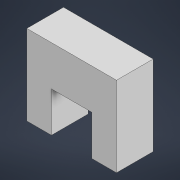
# Autodesk Inventor part: Spacer
Saved by Autodesk Inventor 2022 (Build 260153000, 153)
## iProperties
Created: 2023-04-14
Part Number: Spacer
Material: Všeobecné
Document SubType Name: Modeling
Designer: tada
Density: 1 g/cm^3
Appearance: Výchozí
Author: tada
Autodesk Inventor part; units mm, degrees
ref_plane "YZ Plane" through (0, 0, 0) normal (1, 0, 0) x (0, 1, 0)
ref_plane "XZ Plane" through (0, 0, 0) normal (0, 1, 0) x (-1, 0, 0)
ref_plane "XY Plane" through (0, 0, 0) normal (0, 0, 1) x (1, 0, 0)
sketch "Náčrt1" plane through (0, 0, 0) normal (0, 0, 1) x (1, 0, 0)
  line L0 (7.0986, 0.1592) -> (11.0986, 0.1592)
  line L1 (11.0986, 0.1592) -> (11.0986, 6.6592)
  line L2 (11.0986, 6.6592) -> (17.6486, 6.6592)
  line L3 (17.6486, 6.6592) -> (17.6486, 0.1592)
  line L4 (17.6486, 0.1592) -> (21.6486, 0.1592)
  line L5 (21.6486, 0.1592) -> (21.6486, 13.1592)
  line L6 (21.6486, 13.1592) -> (7.0986, 13.1592)
  line L7 (7.0986, 13.1592) -> (7.0986, 0.1592)
  point P0 (0, 0)
  dimension "d0" = 6.55
  dimension "d1" = 4
  dimension "d2" = 4
  dimension "d3" = 6.5
  dimension "d4" = 13
  constraints: 16 end point, 6 perpendicular, 2 point on line, 1 horizontal
  measures "d0" distance between parallel lines of L1 L3
  measures "d1" distance of L0.start L0.end
  measures "d2" distance of L3.end L4.end
  measures "d3" distance between parallel lines of L2 L0
  measures "d4" distance of L6.end L0.start
extrude "Vysunutí1" add sketch "Náčrt1" along normal blind 5.95
equation "\"d2\" = d1"
